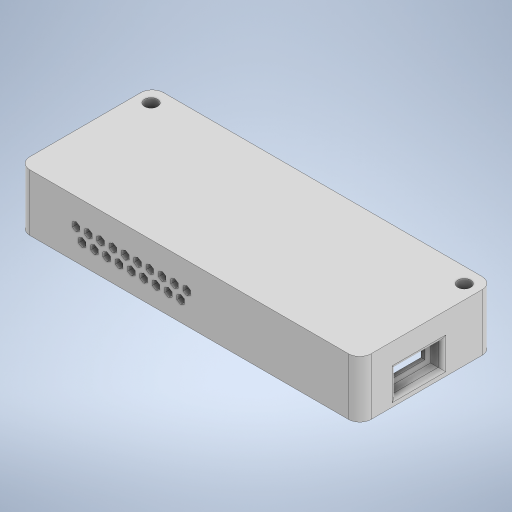
# Autodesk Inventor part: esp32_mount
Saved by Autodesk Inventor 2024 (Build 280153000, 153)
## iProperties
Created: 2024-01-28
Part Number: esp32_mount
Material: Generic
Document SubType Name: Modeling
Designer: crow
Density: 1 g/cm^3
Appearance: Default
Author: crow
## iProperties of the stored document esp32_mount_3DPrint.ipt
Created: 2024-01-28
Part Number: esp32_mount_3DPrint
Material: Generic
Document SubType Name: Modeling
Designer: crow
Density: 1 g/cm^3
Appearance: Default
Author: crow
Autodesk Inventor part; units mm, degrees
ref_plane "YZ Plane" through (0, 0, 0) normal (1, 0, 0) x (0, 1, 0)
ref_plane "XZ Plane" through (0, 0, 0) normal (0, 1, 0) x (-1, 0, 0)
ref_plane "XY Plane" through (0, 0, 0) normal (0, 0, 1) x (1, 0, 0)
sketch "Sketch1" plane through (0, 0, 0) normal (0, 1, 0) x (-1, 0, 0)
  line L0 (-0.1447, 76.4776) -> (-0.1447, -67.7737) construction
  line L1 (44.8553, -21.2084) -> (-45.1447, -21.2084)
  line L2 (-45.1447, -21.2084) -> (-45.1447, -13.2084)
  line L3 (-45.1447, -13.2084) -> (44.8553, -13.2084)
  line L4 (44.8553, -13.2084) -> (44.8553, -21.2084)
  line L5 (40.8553, 10.0416) -> (-41.1447, 10.0416)
  line L6 (-41.1447, 10.0416) -> (-41.1447, -13.2084)
  line L7 (-41.1447, -13.2084) -> (40.8553, -13.2084)
  line L8 (40.8553, -13.2084) -> (40.8553, 10.0416)
  circle A0 centre (7.8763, 7.3066) radius 1.25
  circle A1 centre (7.8763, -10.4734) radius 1.25
  circle A2 centre (-37.8437, -10.4734) radius 1.25
  line L9 (7.8763, 7.3066) -> (7.8763, -10.4734) construction
  line L10 (40.8553, -13.2084) -> (44.8553, -13.2084)
  line L11 (44.8553, -13.2084) -> (44.8553, 14.0416)
  line L12 (44.8553, 14.0416) -> (40.8553, 14.0416)
  line L13 (40.8553, 14.0416) -> (40.8553, -13.2084)
  line L14 (40.8553, 14.0416) -> (-45.1447, 14.0416)
  line L15 (-45.1447, 14.0416) -> (-45.1447, -13.2084)
  circle A3 centre (-37.8437, 7.3066) radius 1.25
  point P0 (0, 0)
  point P1 (41.1603, -17.2084)
  point P2 (-41.4497, -17.2084)
  point P3 (-0.1447, -13.2084)
  point P4 (7.8763, -1.5834)
  point P5 (40.8553, -13.2084)
  dimension "d0" = 82.61
  dimension "d1" = 41.305
  dimension "d2" = 90
  dimension "d3" = 8
  dimension "d4" = 4
  dimension "d5" = 3.695
  dimension "d6" = 82
  dimension "d7" = 23.25
  dimension "d10" = 2.5
  dimension "d11" = 17.78
  dimension "d16" = 43.22
  dimension "d17" = 4
  dimension "d18" = 4
  dimension "d19" = 4
  dimension "d82" = 2.5
  dimension "d85" = 3.301
  dimension "d86" = 45.72
  dimension "d87" = 17.78
  constraints: 32 end point, 6 parallel, 4 centre point, 4 horizontal, 4 perpendicular, 3 midpoint, 2 equal radius, 2 point on line, 2 vertical
  measures "d0" distance of point (41.16, -17.208) point (-41.45, -17.208)
  measures "d1" distance from line of L0 point (-41.45, -17.208)
  measures "d2" distance of L2.end L3.end
  measures "d3" distance of L1.end L2.end
  measures "d4" distance from line of L1 point (-41.45, -17.208)
  measures "d5" distance from line of L2 point (-41.45, -17.208)
  measures "d6" distance of L7.end L6.end
  measures "d7" distance of L6.end L5.end
  measures "d10" diameter of A0
  measures "d11" distance of L9.end L9.start
  measures "d17" distance of L12.end L11.end
  measures "d18" distance between parallel lines of L5 L12
  measures "d19" distance between parallel lines of L6 L15
  measures "d82" diameter of A3
  measures "d85" distance from line of L6 A3.centre
  measures "d86" distance of L9.start A3.centre
  measures "d87" distance of A2.centre A3.centre
extrude "Extrusion1" add sketch "Sketch1" along normal blind 15 contours L1 L2 L3 L4 | L3 L8 L13 L12 L11 | L15 L14 L13 L5 L6 L3
sketch "Sketch2" plane through (0, 15, 0) normal (0, 1, 0) x (1, 0, 0)
  line L0 (-44.8553, 21.2084) -> (-44.8553, -14.0416) construction
  line L1 (-44.8553, 17.2084) -> (45.1447, 17.2084) construction
  line L2 (45.1447, -14.0416) -> (45.1447, 21.2084) construction
  point P0 (0, 0)
  point P1 (-41.1603, 17.2084)
  point P2 (41.4497, 17.2084)
  point P3 (-44.8553, 13.2084)
  point P4 (45.1447, 13.2084)
  dimension "d22" = 82.61
  dimension "d23" = 3.695
  constraints: 3 point on line, 2 end point
  measures "d22" distance of point (-41.16, 17.208) point (41.45, 17.208)
  measures "d23" distance from line of L2 point (41.45, 17.208)
hole "Hole1" at (-41.1603, 15, -17.2084) at (41.4497, 15, -17.2084) direction (0, -1, 0) diameter 3.4 depth 15 clearance for "Countersunk Flat Head Screw ISO 2009/7046" size "M3" standard "ISO"
sketch "Sketch3" plane through (0, 15, 0) normal (0, 1, 0) x (1, 0, 0)
  line L0 (45.1447, 21.2084) -> (-44.8553, 21.2084) projected
  line L1 (-40.8553, 13.2084) -> (41.1447, 13.2084) projected
  line L2 (-44.8553, 21.2084) -> (-29.4803, 21.2084)
  line L3 (-29.4803, 21.2084) -> (-29.4803, 13.2084)
  line L4 (-29.4803, 13.2084) -> (-44.8553, 13.2084)
  line L5 (-44.8553, 13.2084) -> (-44.8553, 21.2084)
  line L6 (-40.8553, 13.2084) -> (41.1447, 13.2084) projected
  line L7 (45.1447, -14.0416) -> (45.1447, 21.2084) projected
  line L8 (29.7697, 13.2084) -> (45.1447, 13.2084)
  line L9 (45.1447, 13.2084) -> (45.1447, 21.2084)
  line L10 (45.1447, 21.2084) -> (29.7697, 21.2084)
  line L11 (29.7697, 21.2084) -> (29.7697, 13.2084)
  circle A0 centre (-41.1603, 17.2084) radius 1.7 projected
  circle A1 centre (-41.1603, 17.2084) radius 3.1
  circle A2 centre (41.4497, 17.2084) radius 1.7 projected
  circle A3 centre (41.4497, 17.2084) radius 3.1
  point P0 (0, 0)
  point P1 (-44.8553, 13.2084)
  point P2 (45.1447, 13.2084)
  point P3 (-44.8553, 13.2084)
  dimension "d72" = 1.4
  dimension "d73" = 1.4
  constraints: 16 end point, 4 parallel, 2 centre point, 2 coincident, 2 horizontal, 2 perpendicular
  measures "d72" radial gap between concentric circles of A1 A0
  measures "d73" radial gap between concentric circles of A3 A2
extrude "Extrusion2" [suppressed]
sketch "Sketch4" plane through (0, 15, 0) normal (0, 1, 0) x (1, 0, 0)
  line L0 (41.1447, -10.0416) -> (-40.8553, -10.0416) projected
  line L1 (41.1447, 13.2084) -> (41.1447, -10.0416) projected
  line L2 (-40.8553, -10.0416) -> (41.1447, -10.0416)
  line L3 (41.1447, -10.0416) -> (41.1447, 13.2084)
  line L4 (41.1447, 13.2084) -> (-40.8553, 13.2084)
  line L5 (-40.8553, 13.2084) -> (-40.8553, -10.0416)
  point P0 (0, 0)
  constraints: 8 end point, 2 parallel, 1 horizontal, 1 perpendicular
extrude "Extrusion3" add sketch "Sketch4" against normal blind 2
sketch "Sketch5" plane through (0, 13, 0) normal (0, -1, 0) x (1, 0, 0)
  circle A0 centre (37.8437, -10.4734) radius 1.25 projected
  circle A1 centre (-7.8763, -10.4734) radius 1.25 projected
  circle A2 centre (-7.8763, 7.3066) radius 1.25 projected
  circle A3 centre (-7.8763, 7.3066) radius 2
  circle A4 centre (-7.8763, -10.4734) radius 2
  circle A5 centre (37.8437, -10.4734) radius 2
  circle A6 centre (37.8437, 7.3066) radius 1.25 projected
  circle A7 centre (37.8437, 7.3066) radius 2
  point P0 (0, 0)
  dimension "d35" = 4
  dimension "d36" = 4
  dimension "d37" = 4
  dimension "d83" = 4
  constraints: 4 centre point, 4 coincident
  measures "d35" diameter of A3
  measures "d36" diameter of A4
  measures "d37" diameter of A5
  measures "d83" diameter of A7
extrude "Extrusion4" add sketch "Sketch5" along normal blind 5 contours A0 | A1 | A2 | A3 | A4 | A5 | A6 | A7
sketch "Sketch6" plane through (37.8437, 8, -10.4734) normal (0, -1, 0) x (1, 0, 0)
  circle A0 centre (0, 0) radius 2 projected
  circle A1 centre (-45.72, 17.78) radius 2 projected
  circle A2 centre (-45.72, 0) radius 2 projected
  circle A3 centre (0, 17.78) radius 2 projected
  point P0 (-37.8437, 10.4734)
  point P1 (-45.72, 17.78)
  point P2 (-45.72, 0)
  point P3 (0, 17.78)
  constraints: 4 coincident
hole "Hole2" at (37.8437, 8, -10.4734) at (-7.8763, 8, 7.3066) at (-7.8763, 8, -10.4734) at (37.8437, 8, 7.3066) direction (0, 1, 0) diameter 2.013 depth 5 thread size "M2.5x0.45" class "6H" standard "ISO Metric profile"
sketch "Sketch7" plane through (45.1447, 0, -13.2084) normal (-1, 0, 0) x (0, 0, 1)
  line L0 (7.085, 3.54) -> (16.225, 3.54)
  line L1 (16.225, 3.54) -> (16.225, 6.95)
  line L2 (16.225, 6.95) -> (7.085, 6.95)
  line L3 (7.085, 6.95) -> (7.085, 3.54)
  line L4 (0, 0) -> (27.25, 0) projected
  line L5 (0, 0) -> (0, 5) projected
  line L6 (27.25, 0) -> (27.25, 15) projected
  line L7 (0, 0) -> (0, 13) projected
  line L8 (27.25, 0) -> (-8, 0) projected
  point P0 (13.2084, 0)
  point P1 (23.25, 0)
  dimension "d53" = 6.95
  dimension "d56" = 7.025
  dimension "d88" = 7.085
  dimension "d89" = 3.54
  constraints: 8 end point, 2 parallel, 1 horizontal, 1 perpendicular
  measures "d53" distance between parallel lines of L4 L2
  measures "d56" distance from line of point (23.25, 0) L1
  measures "d88" distance between parallel lines of L7 L3
  measures "d89" distance between parallel lines of L4 L0
extrude "Extrusion5" cut sketch "Sketch7" along normal blind 5
sketch "Sketch8" plane through (45.1447, 0, -13.2084) normal (-1, 0, 0) x (0, 0, 1)
  line L0 (5.585, 2.04) -> (17.725, 2.04)
  line L1 (17.725, 2.04) -> (17.725, 8.45)
  line L2 (17.725, 8.45) -> (5.585, 8.45)
  line L3 (5.585, 8.45) -> (5.585, 2.04)
  line L4 (16.225, 6.95) -> (16.225, 3.54) projected
  line L5 (7.085, 3.54) -> (7.085, 6.95) projected
  line L6 (16.225, 3.54) -> (7.085, 3.54) projected
  line L7 (7.085, 6.95) -> (16.225, 6.95) projected
  point P0 (13.2084, 0)
  dimension "d58" = 1.5
  dimension "d59" = 1.5
  dimension "d60" = 1.5
  dimension "d61" = 1.5
  constraints: 8 end point, 2 parallel, 1 horizontal, 1 perpendicular
  measures "d58" distance between parallel lines of L1 L4
  measures "d59" distance between parallel lines of L3 L5
  measures "d60" distance between parallel lines of L0 L6
  measures "d61" distance between parallel lines of L2 L7
extrude "Extrusion6" cut sketch "Sketch8" along normal blind 3 contours L3 L2 L1 L0 | L4 L6 L5 L7
fillet "Fillet2" radius 1 4 edges at (45.1447, 5.245, -7.6234) (45.1447, 2.04, -1.5534) (45.1447, 8.45, -1.5534) (45.1447, 5.245, 4.5166)
sketch "Sketch9" plane through (-44.8553, 0, 14.0416) normal (0, 0, 1) x (1, 0, 0)
  line L0 (39.5056, 7.1579) -> (41.1292, 6.2205)
  line L1 (41.1292, 6.2205) -> (41.1292, 4.3457)
  line L2 (41.1292, 4.3457) -> (39.5056, 3.4083)
  line L3 (39.5056, 3.4083) -> (37.882, 4.3457)
  line L4 (37.882, 4.3457) -> (37.882, 6.2205)
  line L5 (37.882, 6.2205) -> (39.5056, 7.1579)
  line L6 (39.5056, 7.1579) -> (39.5056, 9.0326)
  line L7 (39.5056, 9.0326) -> (37.882, 9.97)
  line L8 (37.882, 9.97) -> (36.2584, 9.0326)
  line L9 (36.2584, 9.0326) -> (36.2584, 7.1579)
  line L10 (36.2584, 7.1579) -> (37.882, 6.2205)
  line L11 (37.882, 6.2205) -> (37.882, 4.3457)
  line L12 (34.6348, 4.3457) -> (34.6348, 6.2205)
  line L13 (36.2584, 3.4083) -> (34.6348, 4.3457)
  line L14 (37.882, 4.3457) -> (36.2584, 3.4083)
  line L15 (34.6348, 6.2205) -> (36.2584, 7.1579)
  line L16 (34.6348, 9.97) -> (36.2584, 9.0326)
  line L17 (36.2584, 7.1579) -> (36.2584, 9.0326)
  line L18 (34.6348, 9.97) -> (33.0112, 9.0326)
  line L19 (33.0112, 9.0326) -> (33.0112, 7.1579)
  line L20 (33.0112, 7.1579) -> (34.6348, 6.2205)
  line L21 (33.0112, 3.4083) -> (34.6348, 4.3457)
  line L22 (34.6348, 6.2205) -> (34.6348, 4.3457)
  line L23 (31.3876, 4.3457) -> (31.3876, 6.2205)
  line L24 (31.3876, 4.3457) -> (33.0112, 3.4083)
  line L25 (31.3876, 6.2205) -> (33.0112, 7.1579)
  line L26 (31.3876, 9.97) -> (33.0112, 9.0326)
  line L27 (33.0112, 7.1579) -> (33.0112, 9.0326)
  line L28 (29.764, 7.1579) -> (29.764, 9.0326)
  line L29 (29.764, 7.1579) -> (31.3876, 6.2205)
  line L30 (29.764, 9.0326) -> (31.3876, 9.97)
  line L31 (39.5056, 6.4378) -> (40.5056, 5.8604)
  line L32 (40.5056, 5.8604) -> (40.5056, 4.7057)
  line L33 (40.5056, 4.7057) -> (39.5056, 4.1284)
  line L34 (39.5056, 4.1284) -> (38.5056, 4.7057)
  line L35 (38.5056, 4.7057) -> (38.5056, 5.8604)
  line L36 (38.5056, 5.8604) -> (39.5056, 6.4378)
  line L37 (36.2584, 6.4378) -> (35.2584, 5.8604)
  line L38 (35.2584, 5.8604) -> (35.2584, 4.7057)
  line L39 (35.2584, 4.7057) -> (36.2584, 4.1284)
  line L40 (36.2584, 4.1284) -> (37.2584, 4.7057)
  line L41 (37.2584, 4.7057) -> (37.2584, 5.8604)
  line L42 (37.2584, 5.8604) -> (36.2584, 6.4378)
  line L43 (33.0112, 6.4378) -> (34.0112, 5.8604)
  line L44 (32.0112, 5.8604) -> (33.0112, 6.4378)
  line L45 (32.0112, 4.7057) -> (32.0112, 5.8604)
  line L46 (34.0112, 5.8604) -> (34.0112, 4.7057)
  line L47 (34.0112, 4.7057) -> (33.0112, 4.1284)
  line L48 (33.0112, 4.1284) -> (32.0112, 4.7057)
  line L49 (33.6348, 8.6726) -> (33.6348, 7.5179)
  line L50 (33.6348, 7.5179) -> (34.6348, 6.9406)
  line L51 (34.6348, 9.25) -> (33.6348, 8.6726)
  line L52 (34.6348, 6.9406) -> (35.6348, 7.5179)
  line L53 (35.6348, 8.6726) -> (34.6348, 9.25)
  line L54 (35.6348, 7.5179) -> (35.6348, 8.6726)
  line L55 (32.3876, 8.6726) -> (32.3876, 7.5179)
  line L56 (32.3876, 7.5179) -> (31.3876, 6.9406)
  line L57 (31.3876, 9.25) -> (32.3876, 8.6726)
  line L58 (30.3876, 8.6726) -> (31.3876, 9.25)
  line L59 (31.3876, 6.9406) -> (30.3876, 7.5179)
  line L60 (30.3876, 7.5179) -> (30.3876, 8.6726)
  line L61 (38.882, 8.6726) -> (38.882, 7.5179)
  line L62 (38.882, 7.5179) -> (37.882, 6.9406)
  line L63 (37.882, 9.25) -> (38.882, 8.6726)
  line L64 (36.882, 8.6726) -> (37.882, 9.25)
  line L65 (37.882, 6.9406) -> (36.882, 7.5179)
  line L66 (36.882, 7.5179) -> (36.882, 8.6726)
  line L67 (41.1292, 6.2205) -> (42.7528, 7.1579)
  line L68 (42.7528, 7.1579) -> (42.7528, 9.0326)
  line L69 (42.7528, 9.0326) -> (41.1292, 9.97)
  line L70 (41.1292, 9.97) -> (39.5056, 9.0326)
  line L71 (39.5056, 9.0326) -> (39.5056, 7.1579)
  line L72 (40.1292, 7.5179) -> (41.1292, 6.9406)
  line L73 (41.1292, 6.9406) -> (42.1292, 7.5179)
  line L74 (42.1292, 7.5179) -> (42.1292, 8.6726)
  line L75 (42.1292, 8.6726) -> (41.1292, 9.25)
  line L76 (41.1292, 9.25) -> (40.1292, 8.6726)
  line L77 (40.1292, 8.6726) -> (40.1292, 7.5179)
  line L78 (41.1292, 4.3457) -> (41.1292, 6.2205)
  line L79 (41.1292, 4.3457) -> (42.7528, 3.4083)
  line L80 (42.7528, 4.1284) -> (41.7528, 4.7057)
  line L81 (43.7528, 4.7057) -> (42.7528, 4.1284)
  line L82 (43.7528, 5.8604) -> (43.7528, 4.7057)
  line L83 (44.3764, 6.2205) -> (44.3764, 4.3457)
  line L84 (42.7528, 6.4378) -> (43.7528, 5.8604)
  line L85 (41.7528, 5.8604) -> (42.7528, 6.4378)
  line L86 (41.7528, 4.7057) -> (41.7528, 5.8604)
  line L87 (42.7528, 7.1579) -> (44.3764, 6.2205)
  line L88 (44.3764, 4.3457) -> (42.7528, 3.4083)
  line L89 (42.7528, 9.0326) -> (44.3764, 9.97)
  line L90 (42.7528, 9.0326) -> (42.7528, 7.1579)
  line L91 (45.3764, 7.5179) -> (45.3764, 8.6726)
  line L92 (44.3764, 9.25) -> (43.3764, 8.6726)
  line L93 (44.3764, 6.9406) -> (45.3764, 7.5179)
  line L94 (43.3764, 8.6726) -> (43.3764, 7.5179)
  line L95 (43.3764, 7.5179) -> (44.3764, 6.9406)
  line L96 (44.3764, 6.2205) -> (46, 7.1579)
  line L97 (45.3764, 8.6726) -> (44.3764, 9.25)
  line L98 (44.3764, 9.97) -> (46, 9.0326)
  line L99 (46, 7.1579) -> (46, 9.0326)
  line L100 (90, 0) -> (90, 15) projected
  line L101 (23.2695, 7.1579) -> (24.8931, 6.2205)
  line L102 (24.8931, 6.2205) -> (24.8931, 4.3457)
  line L103 (24.8931, 4.3457) -> (23.2695, 3.4083)
  line L104 (23.2695, 3.4083) -> (21.6459, 4.3457)
  line L105 (21.6459, 4.3457) -> (21.6459, 6.2205)
  line L106 (21.6459, 6.2205) -> (23.2695, 7.1579)
  line L107 (21.6459, 9.97) -> (20.0223, 9.0326)
  line L108 (23.2695, 9.0326) -> (21.6459, 9.97)
  line L109 (23.2695, 7.1579) -> (23.2695, 9.0326)
  line L110 (20.0223, 7.1579) -> (21.6459, 6.2205)
  line L111 (20.0223, 9.0326) -> (20.0223, 7.1579)
  line L112 (21.6459, 4.3457) -> (20.0223, 3.4083)
  line L113 (20.0223, 3.4083) -> (18.3987, 4.3457)
  line L114 (18.3987, 4.3457) -> (18.3987, 6.2205)
  line L115 (18.3987, 6.2205) -> (20.0223, 7.1579)
  line L116 (21.6459, 6.2205) -> (21.6459, 4.3457)
  line L117 (18.3987, 9.97) -> (16.7751, 9.0326)
  line L118 (18.3987, 9.97) -> (20.0223, 9.0326)
  line L119 (20.0223, 7.1579) -> (20.0223, 9.0326)
  line L120 (16.7751, 7.1579) -> (18.3987, 6.2205)
  line L121 (16.7751, 9.0326) -> (16.7751, 7.1579)
  line L122 (15.1515, 4.3457) -> (16.7751, 3.4083)
  line L123 (15.1515, 4.3457) -> (15.1515, 6.2205)
  line L124 (15.1515, 6.2205) -> (16.7751, 7.1579)
  line L125 (18.3987, 6.2205) -> (18.3987, 4.3457)
  line L126 (16.7751, 3.4083) -> (18.3987, 4.3457)
  line L127 (16.7751, 7.1579) -> (16.7751, 9.0326)
  line L128 (13.5279, 9.0326) -> (15.1515, 9.97)
  line L129 (13.5279, 7.1579) -> (13.5279, 9.0326)
  line L130 (13.5279, 7.1579) -> (15.1515, 6.2205)
  line L131 (15.1515, 9.97) -> (16.7751, 9.0326)
  line L132 (23.2695, 6.4378) -> (24.2695, 5.8604)
  line L133 (24.2695, 5.8604) -> (24.2695, 4.7057)
  line L134 (24.2695, 4.7057) -> (23.2695, 4.1284)
  line L135 (23.2695, 4.1284) -> (22.2695, 4.7057)
  line L136 (22.2695, 4.7057) -> (22.2695, 5.8604)
  line L137 (22.2695, 5.8604) -> (23.2695, 6.4378)
  line L138 (20.0223, 6.4378) -> (19.0223, 5.8604)
  line L139 (21.0223, 5.8604) -> (20.0223, 6.4378)
  line L140 (21.0223, 4.7057) -> (21.0223, 5.8604)
  line L141 (19.0223, 5.8604) -> (19.0223, 4.7057)
  line L142 (19.0223, 4.7057) -> (20.0223, 4.1284)
  line L143 (20.0223, 4.1284) -> (21.0223, 4.7057)
  line L144 (15.7751, 5.8604) -> (16.7751, 6.4378)
  line L145 (16.7751, 6.4378) -> (17.7751, 5.8604)
  line L146 (15.7751, 4.7057) -> (15.7751, 5.8604)
  line L147 (17.7751, 5.8604) -> (17.7751, 4.7057)
  line L148 (16.7751, 4.1284) -> (15.7751, 4.7057)
  line L149 (17.7751, 4.7057) -> (16.7751, 4.1284)
  line L150 (17.3987, 8.6726) -> (17.3987, 7.5179)
  line L151 (17.3987, 7.5179) -> (18.3987, 6.9406)
  line L152 (18.3987, 9.25) -> (17.3987, 8.6726)
  line L153 (19.3987, 8.6726) -> (18.3987, 9.25)
  line L154 (18.3987, 6.9406) -> (19.3987, 7.5179)
  line L155 (19.3987, 7.5179) -> (19.3987, 8.6726)
  line L156 (16.1515, 7.5179) -> (15.1515, 6.9406)
  line L157 (15.1515, 6.9406) -> (14.1515, 7.5179)
  line L158 (16.1515, 8.6726) -> (16.1515, 7.5179)
  line L159 (15.1515, 9.25) -> (16.1515, 8.6726)
  line L160 (14.1515, 7.5179) -> (14.1515, 8.6726)
  line L161 (14.1515, 8.6726) -> (15.1515, 9.25)
  line L162 (22.6459, 7.5179) -> (21.6459, 6.9406)
  line L163 (21.6459, 6.9406) -> (20.6459, 7.5179)
  line L164 (22.6459, 8.6726) -> (22.6459, 7.5179)
  line L165 (21.6459, 9.25) -> (22.6459, 8.6726)
  line L166 (20.6459, 7.5179) -> (20.6459, 8.6726)
  line L167 (20.6459, 8.6726) -> (21.6459, 9.25)
  line L168 (23.8931, 8.6726) -> (23.8931, 7.5179)
  line L169 (23.2695, 9.0326) -> (23.2695, 7.1579)
  line L170 (24.8931, 9.25) -> (23.8931, 8.6726)
  line L171 (25.8931, 8.6726) -> (24.8931, 9.25)
  line L172 (26.5167, 9.0326) -> (24.8931, 9.97)
  line L173 (25.8931, 7.5179) -> (25.8931, 8.6726)
  line L174 (24.8931, 6.9406) -> (25.8931, 7.5179)
  line L175 (23.8931, 7.5179) -> (24.8931, 6.9406)
  line L176 (26.5167, 7.1579) -> (26.5167, 9.0326)
  line L177 (24.8931, 6.2205) -> (26.5167, 7.1579)
  line L178 (24.8931, 9.97) -> (23.2695, 9.0326)
  line L179 (27.5167, 4.7057) -> (26.5167, 4.1284)
  line L180 (25.5167, 4.7057) -> (25.5167, 5.8604)
  line L181 (27.5167, 5.8604) -> (27.5167, 4.7057)
  line L182 (25.5167, 5.8604) -> (26.5167, 6.4378)
  line L183 (26.5167, 6.4378) -> (27.5167, 5.8604)
  line L184 (28.1404, 6.2205) -> (28.1404, 4.3457)
  line L185 (26.5167, 7.1579) -> (28.1404, 6.2205)
  line L186 (26.5167, 4.1284) -> (25.5167, 4.7057)
  line L187 (24.8931, 4.3457) -> (26.5167, 3.4083)
  line L188 (28.1404, 4.3457) -> (26.5167, 3.4083)
  line L189 (24.8931, 4.3457) -> (24.8931, 6.2205)
  line L190 (26.5167, 9.0326) -> (26.5167, 7.1579)
  line L191 (27.1404, 8.6726) -> (27.1404, 7.5179)
  line L192 (27.1404, 7.5179) -> (28.1404, 6.9406)
  line L193 (29.1404, 8.6726) -> (28.1404, 9.25)
  line L194 (28.1404, 6.9406) -> (29.1404, 7.5179)
  line L195 (28.1404, 9.97) -> (29.764, 9.0326)
  line L196 (29.1404, 7.5179) -> (29.1404, 8.6726)
  line L197 (28.1404, 6.2205) -> (29.764, 7.1579)
  line L198 (29.764, 7.1579) -> (29.764, 9.0326)
  line L199 (26.5167, 9.0326) -> (28.1404, 9.97)
  line L200 (28.1404, 9.25) -> (27.1404, 8.6726)
  line L201 (28.1404, 4.3457) -> (28.1404, 6.2205)
  line L202 (29.764, 7.1579) -> (28.1404, 6.2205)
  line L203 (31.3876, 4.3457) -> (29.764, 3.4083)
  line L204 (31.3876, 6.2205) -> (29.764, 7.1579)
  line L205 (29.764, 3.4083) -> (28.1404, 4.3457)
  line L206 (33.0112, 7.1579) -> (31.3876, 6.2205)
  line L207 (30.764, 5.8604) -> (29.764, 6.4378)
  line L208 (29.764, 6.4378) -> (28.764, 5.8604)
  line L209 (30.764, 4.7057) -> (30.764, 5.8604)
  line L210 (28.764, 5.8604) -> (28.764, 4.7057)
  line L211 (29.764, 4.1284) -> (30.764, 4.7057)
  line L212 (28.764, 4.7057) -> (29.764, 4.1284)
  point P0 (44.8553, 0)
  point P1 (39.5056, 5.2831)
  point P2 (39.5056, 5.2831)
  point P3 (36.2584, 5.2831)
  point P4 (36.2584, 5.2831)
  point P5 (33.0112, 5.2831)
  point P6 (33.0112, 5.2831)
  point P7 (34.6348, 8.0953)
  point P8 (34.6348, 8.0953)
  point P9 (31.3876, 8.0953)
  point P10 (31.3876, 8.0953)
  point P11 (37.882, 8.0953)
  point P12 (37.882, 8.0953)
  point P13 (31.3876, 5.2831)
  point P14 (41.1292, 8.0953)
  point P15 (41.1292, 8.0953)
  point P16 (42.7528, 5.2831)
  point P17 (42.7528, 5.2831)
  point P18 (44.3764, 8.0953)
  point P19 (44.3764, 8.0953)
  point P20 (43.7528, 5.2831)
  point P21 (23.2695, 5.2831)
  point P22 (23.2695, 5.2831)
  point P23 (20.0223, 5.2831)
  point P24 (20.0223, 5.2831)
  point P25 (16.7751, 5.2831)
  point P26 (16.7751, 5.2831)
  point P27 (18.3987, 8.0953)
  point P28 (18.3987, 8.0953)
  point P29 (15.1515, 8.0953)
  point P30 (15.1515, 8.0953)
  point P31 (21.6459, 8.0953)
  point P32 (21.6459, 8.0953)
  point P33 (15.1515, 5.2831)
  point P34 (24.8931, 8.0953)
  point P35 (24.8931, 8.0953)
  point P36 (26.5167, 5.2831)
  point P37 (26.5167, 5.2831)
  point P38 (28.1404, 8.0953)
  point P39 (28.1404, 8.0953)
  point P40 (27.5167, 5.2831)
  point P41 (29.764, 5.2831)
  point P42 (29.764, 5.2831)
  dimension "d68" = 2
  dimension "d69" = 3.2472
  dimension "d74" = 44
  dimension "d76" = 2
  dimension "d77" = 3.2472
  dimension "d79" = 0
  dimension "d80" = 0
  constraints: 424 end point, 189 symmetric about line, 19 coincident, 4 midpoint, 52 other
  measures "d68" distance from line of point (43.753, 5.283) L86
  measures "d69" distance between parallel lines of L1 L83
  measures "d74" distance between parallel lines of L100 L99
  measures "d76" distance from line of point (27.517, 5.283) L180
  measures "d77" distance between parallel lines of L102 L184
  measures "d79" distance between parallel lines of L28 L198
  measures "d80" distance of L30.start L195.end
extrude "Extrusion7" cut sketch "Sketch9" against normal up to surface (4 mm away) contours L31 L32 L33 L34 L35 L36 | L42 L41 L40 L39 L38 L37 | L43 L46 L47 L48 L45 L44 | L51 L53 L54 L52 L50 L49 | L55 L56 L59 L60 L58 L57 | L61 L62 L65 L66 L64 L63 | L77 L76 L75 L74 L73 L72 | L80 L86 L85 L84 L82 L81 | L93 L95 L94 L92 L97 L91 | L132 L133 L134 L135 L136 L137 | L139 L140 L143 L142 L141 L138 | L144 L145 L147 L149 L148 L146 | L152 L153 L155 L154 L151 L150 | L156 L157 L160 L161 L159 L158 | L162 L163 L166 L167 L165 L164 | L170 L171 L173 L174 L175 L168 | L179 L186 L180 L182 L183 L181 | L200 L193 L196 L194 L192 L191 | L209 L211 L212 L210 L208 L207
fillet "Fillet3" radius 3 4 edges at (45.1447, 7.5, -21.2084) (45.1447, 7.5, 14.0416) (-44.8553, 7.5, 14.0416) (-44.8553, 7.5, -21.2084)
equation "\"d73\" = d72"
equation "\"d36\" = d35"
equation "\"d37\" = d35"
equation "\"d83\" = d35"
equation "\"d59\" = d58"
equation "\"d60\" = d58"
equation "\"d61\" = d58"
body "Solid189"
